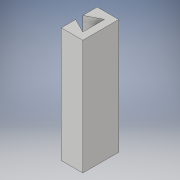
# Autodesk Inventor part: Part2
Saved by Autodesk Inventor 2018.2 (Build 222227000, 227)
## iProperties
Created: 2018-03-30
Part Number: Part2
Material: Generic
Document SubType Name: Modeling
Designer: martin
Density: 1 g/cm^3
Appearance: Default
Author: martin
Autodesk Inventor part; units mm, degrees
ref_plane "YZ Plane" through (0, 0, 0) normal (1, 0, 0) x (0, 1, 0)
ref_plane "XZ Plane" through (0, 0, 0) normal (0, 1, 0) x (-1, 0, 0)
ref_plane "XY Plane" through (0, 0, 0) normal (0, 0, 1) x (1, 0, 0)
sketch "Sketch2" plane through (0, 0, 0) normal (0, 1, 0) x (-1, 0, 0)
  line L0 (0, 0) -> (0, -7.9375)
  line L1 (0, -7.9375) -> (9.525, -7.9375)
  line L2 (9.525, -7.9375) -> (9.525, -1.5875)
  line L3 (9.525, -1.5875) -> (3.175, -4.7625)
  line L4 (3.175, -4.7625) -> (3.175, 0)
  line L5 (3.175, 0) -> (0, 0)
  line L6 (0, 0) -> (0, 7.9375)
  line L7 (0, 7.9375) -> (9.525, 7.9375)
  line L8 (9.525, 7.9375) -> (9.525, 1.5875)
  line L9 (9.525, 1.5875) -> (3.175, 4.7625)
  line L10 (3.175, 4.7625) -> (3.175, 0)
  dimension "d1" = 7.9375
  dimension "d2" = 9.525
  dimension "d3" = 6.35
  dimension "d4" = 4.7625
  dimension "d5" = 3.175
  constraints: 22 end point, 4 symmetric about line, 2 parallel, 2 perpendicular, 1 vertical
  measures "d1" distance of L0.start L0.end
  measures "d2" distance of L0.end L1.end
  measures "d3" distance of L1.end L2.end
  measures "d4" distance of L3.end L4.end
  measures "d5" distance of L4.end L0.start
extrude "Extrusion1" add sketch "Sketch2" along normal mid plane 50.8
body "Solid1"
